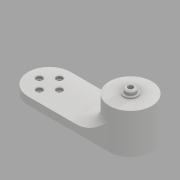
# Autodesk Inventor part: Arm - right actuator hinge
Saved by Autodesk Inventor 2017 (Build 210142000, 142)
## iProperties
Created: 2016-03-31
Part Number: Arm - right actuator hinge
Material: Generic
Document SubType Name: Modeling
Designer: alist
Density: 1 g/cm^3
Appearance: Default
Author: alist
## iProperties of the stored document Arm - actuator hinge R_3DPrint.ipt
Created: 2017-04-11
Part Number: Arm - actuator hinge R_3DPrint
Material: Generic
Document SubType Name: Modeling
Designer: Ali
Density: 1 g/cm^3
Appearance: Default
Author: Ali
Autodesk Inventor part; units mm, degrees
ref_plane "YZ Plane" through (0, 0, 0) normal (1, 0, 0) x (0, 1, 0)
ref_plane "XZ Plane" through (0, 0, 0) normal (0, 1, 0) x (-1, 0, 0)
ref_plane "XY Plane" through (0, 0, 0) normal (0, 0, 1) x (1, 0, 0)
sketch "Sketch1" plane through (0, 0, 0) normal (0, 0, 1) x (1, 0, 0)
  line L0 (-32.5, 0) -> (32.5, 0) construction
  line L1 (-32.5, -17) -> (32.5, -17)
  line L2 (32.5, 17) -> (-32.5, 17)
  arc A0 (-32.5, 17) -> (-32.5, -17) centre (-32.5, 0) ccw
  arc A1 (32.5, -17) -> (32.5, 17) centre (32.5, 0) ccw
  point P0 (0, 0)
  point P1 (0, 0)
  dimension "d1" = 65
  dimension "d2" = 34
  constraints: 8 end point, 4 point on circle, 4 tangent, 2 centre point, 1 coincident, 1 horizontal, 1 midpoint, 1 parallel
  measures "d1" distance of L0.start L0.end
  measures "d2" diameter of A1
extrude "Extrusion1" add sketch "Sketch1" along normal blind 6
sketch "Sketch2" plane through (0, 0, 6) normal (0, 0, 1) x (1, 0, 0)
  arc A0 (32.5, -17) -> (32.5, 17) centre (32.5, 0) ccw projected
  circle A1 centre (32.5, 0) radius 17
  point P0 (0, 0)
  constraints: 1 coincident, 1 vertical alignment, 2 other
extrude "Extrusion2" add sketch "Sketch2" along normal blind 26
sketch "Sketch3" plane through (0, 0, 0) normal (0, 0, -1) x (-1, 0, 0)
  arc A0 (32.5, -17) -> (32.5, 17) centre (32.5, 0) ccw projected
  circle A1 centre (32.5, 0) radius 8 construction
  circle A2 centre (32.5, 8) radius 1.2
  circle A3 centre (24.5, 0) radius 1.2
  circle A4 centre (32.5, -8) radius 1.2
  circle A5 centre (40.5, 0) radius 1.2
  point P0 (0, 0)
  dimension "d7" = 16
  dimension "d8" = 2.4
  dimension "d11" = 360
  constraints: 4 centre point, 1 coincident, 1 vertical alignment, 11 other
  measures "d8" diameter of A2
extrude "Extrusion3" cut sketch "Sketch3" against normal through all
sketch "Sketch4" plane through (0, 0, 6) normal (0, 0, 1) x (1, 0, 0)
  circle A0 centre (-32.5, 8) radius 1.2 projected
  circle A1 centre (-24.5, 0) radius 1.2 projected
  circle A2 centre (-32.5, -8) radius 1.2 projected
  circle A3 centre (-40.5, 0) radius 1.2 projected
  circle A4 centre (-32.5, 8) radius 2.5
  circle A5 centre (-24.5, 0) radius 2.5
  circle A6 centre (-32.5, -8) radius 2.5
  circle A7 centre (-40.5, 0) radius 2.5
  point P0 (0, 0)
  dimension "d15" = 5
  dimension "d16" = 5
  dimension "d17" = 5
  dimension "d18" = 5
  constraints: 4 centre point, 4 coincident
  measures "d15" diameter of A4
  measures "d16" diameter of A5
  measures "d17" diameter of A6
  measures "d18" diameter of A7
extrude "Extrusion4" cut sketch "Sketch4" against normal blind 2
sketch "Sketch5" plane through (0, 0, 0) normal (0, 0, -1) x (-1, 0, 0)
  arc A0 (-32.5, 13) -> (-32.5, -13) centre (-32.5, 0) ccw projected
  circle A1 centre (-32.5, 0) radius 7.5
  point P0 (0, 0)
  dimension "d22" = 15
  constraints: 1 centre point, 1 coincident
  measures "d22" diameter of A1
extrude "Extrusion5" cut sketch "Sketch5" against normal blind 18
sketch "Sketch6" plane through (32.5, 0, 18) normal (0, 0, -1) x (-1, 0, 0)
  line L0 (0.0156, 4.1569) -> (3.6078, 2.0649)
  line L1 (3.6078, 2.0649) -> (3.5922, -2.092)
  line L2 (3.5922, -2.092) -> (-0.0156, -4.1569)
  line L3 (-0.0156, -4.1569) -> (-3.6078, -2.0649)
  line L4 (-3.6078, -2.0649) -> (-3.5922, 2.092)
  line L5 (-3.5922, 2.092) -> (0.0156, 4.1569)
  point P0 (32.5, 0)
  point P1 (0, 0)
  dimension "d26" = 7.2
  constraints: 12 end point, 13 other
  measures "d26" distance between parallel lines of L1 L4
extrude "Extrusion6" cut sketch "Sketch6" against normal blind 3.5
sketch "Sketch7" plane through (32.5, 0, 32) normal (0, 0, 1) x (1, 0, 0)
  circle A0 centre (0, 0) radius 5.5
  point P0 (-32.5, 0)
  dimension "d29" = 11
  constraints: 1 centre point
  measures "d29" diameter of A0
extrude "Extrusion7" add sketch "Sketch7" along normal blind 1
sketch "Sketch8" plane through (32.5, 0, 33) normal (0, 0, 1) x (1, 0, 0)
  circle A0 centre (0, 0) radius 4
  point P0 (-32.5, 0)
  dimension "d32" = 8
  constraints: 1 centre point
  measures "d32" diameter of A0
extrude "Extrusion8" add sketch "Sketch8" along normal blind 3.5
chamfer "Chamfer1" distance 1 angle 45 1 edges at (28.5, 0, 36.5)
hole "Hole1" at (32.5, 0, 36.5) direction (0, 0, -1) diameter 4.3 end through all
chamfer "Chamfer2" distance 2 angle 45 1 edges at (32.5, 2.15, 21.5)
fillet "Fillet3" radius 15 1 edges at (15.5, 0, 6)
chamfer "Chamfer3" distance 3.9 angle 45 1 edges at (40, 0, 18)
body "Solid1"
